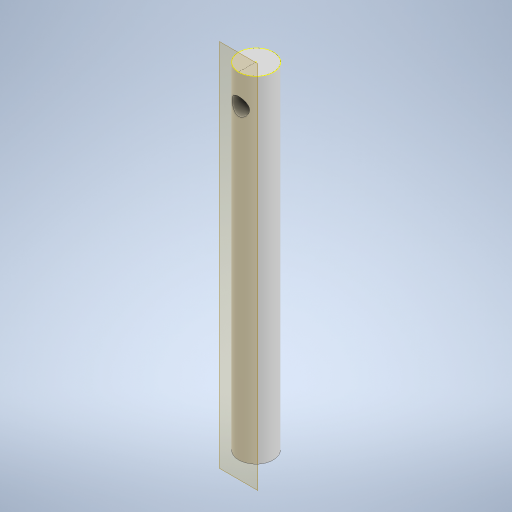
# Autodesk Inventor part: 16_Soporte
Saved by Autodesk Inventor 2024.2 (Build 282272000, 272)
## iProperties
Created: 2024-04-26
Part Number: 16_Soporte
Material: Genérico
Document SubType Name: Modeling
Designer: Cosmic Dinodog
Density: 1 g/cm^3
Appearance: Valor por defecto
Author: Cosmic Dinodog
Autodesk Inventor part; units mm, degrees
ref_plane "YZ Plane" through (0, 0, 0) normal (1, 0, 0) x (0, 1, 0)
ref_plane "XZ Plane" through (0, 0, 0) normal (0, 1, 0) x (-1, 0, 0)
sketch "Boceto1" plane through (0, 0, 0) normal (0, 1, 0) x (-1, 0, 0)
  circle A0 centre (0, 0) radius 7
  dimension "d0" = 14
  constraints: 1 centre point, 1 coincident
  measures "d0" diameter of A0
extrude "Extrusión1" add sketch "Boceto1" along normal blind 135.5
sketch "Boceto2" plane through (0, 135.5, 0) normal (0, 1, 0) x (1, 0, 0)
  line L0 (0, 0) -> (0, -7) construction
  circle A0 centre (0, 0) radius 7 projected
  constraints: 2 end point, 1 vertical, 1 vertical alignment, 1 other
ref_plane "Plano de trabajo1" through (0, 135.5, 7) normal (0, 0, 1) x (1, 0, 0)
sketch "Boceto3" plane through (0, 135.5, 7) normal (0, 0, 1) x (1, 0, 0)
  line L0 (7, 0) -> (-7, 0) construction
  line L1 (0, 0) -> (0, -12) construction
  circle A0 centre (0, -12) radius 3.5
  point P0 (0, -135.5)
  dimension "d3" = 12
  dimension "d4" = 7
  constraints: 2 end point, 1 centre point, 1 coincident, 1 midpoint, 1 vertical
  measures "d3" distance of L1.start L1.end
  measures "d4" diameter of A0
hole "Agujero1" at (0, 123.5, 7) direction (0, 0, -1) diameter 7 end through all
